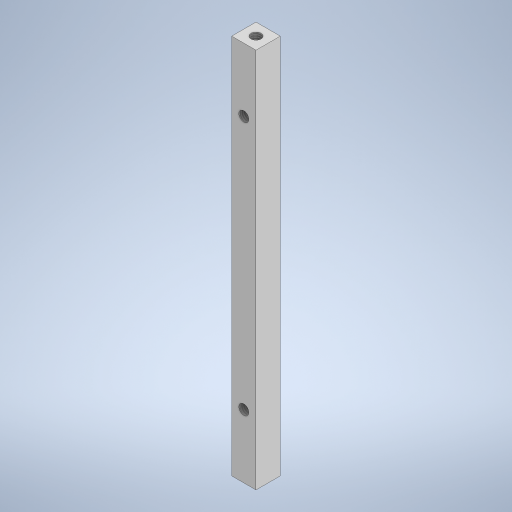
# Autodesk Inventor part: VerticalStrut
Saved by Autodesk Inventor 2023 (Build 270158000, 158)
## iProperties
Created: 2022-07-23
Part Number: VerticalStrut
Material: Generic
Document SubType Name: Modeling
Designer: Aditya Bansal
Density: 1 g/cm^3
Appearance: Default
Author: Aditya Bansal
Autodesk Inventor part; units mm, degrees
ref_plane "YZ Plane" through (0, 0, 0) normal (1, 0, 0) x (0, 1, 0)
ref_plane "XZ Plane" through (0, 0, 0) normal (0, 1, 0) x (-1, 0, 0)
ref_plane "XY Plane" through (0, 0, 0) normal (0, 0, 1) x (1, 0, 0)
sketch "Sketch1" plane through (0, 0, 0) normal (0, 1, 0) x (-1, 0, 0)
  line L0 (0, 0) -> (6, 0)
  line L1 (6, 0) -> (6, -6)
  line L2 (6, -6) -> (0, -6)
  line L3 (0, -6) -> (0, 0)
  dimension "d0" = 6
  constraints: 8 end point, 2 parallel, 2 perpendicular, 1 horizontal
  measures "d0" distance of L0.end L1.end
extrude "Extrusion1" add sketch "Sketch1" along normal blind 47
sketch "Sketch2" plane through (0, 47, 0) normal (0, 1, 0) x (1, 0, 0)
  line L0 (0, 6) -> (-6, 6) projected
  line L1 (0, 0) -> (0, 6) projected
  point P0 (-3, 3)
  point P1 (-3, 6)
  point P2 (0, 3)
  point P3 (-3, 6)
  constraints: 3 midpoint, 1 horizontal alignment, 1 vertical alignment
hole "Hole1" at (-3, 47, -3) direction (0, -1, 0) diameter 2.459 depth 10 tip angle 118 thread size "M3x0.5" class "6H" standard "ANSI Metric M Profile"
sketch "Sketch3" plane through (-6, 47, 0) normal (0, 0, 1) x (1, 0, 0)
  line L0 (0, -47) -> (0, 0) projected
  line L1 (6, -47) -> (6, 0) projected
  line L2 (0, 0) -> (6, 0) projected
  point P0 (3, -47)
  point P1 (3, -15.6667)
  point P2 (0, -94)
  point P3 (6, -94)
  dimension "d17" = 6
  dimension "d18" = 3
  dimension "d19" = 15.6667
  dimension "d20" = 31.3333
  dimension "d21" = 47
  constraints: 1 point on line, 1 vertical alignment
  measures "d17" distance between parallel lines of L0 L1
  measures "d18" distance from line of L1 point (3, -15.667)
  measures "d19" distance from line of point (3, -15.667) L2
  measures "d20" distance of point (3, -15.667) point (3, -47)
  measures "d21" distance from line of L2 point (6, -47)
hole "Hole2" at (-3, 31.3333, 0) direction (0, 0, -1) diameter 2.459 depth 3 tip angle 118 thread size "M3x0.5" class "6H" standard "ANSI Metric M Profile"
sketch "Sketch5" plane through (-6, 0, -6) normal (-1, 0, 0) x (0, 0, 1)
  line L0 (0, 0) -> (6, 0) projected
  point P0 (3, 25)
  point P1 (3, 0)
  dimension "d29" = 25
  constraints: 1 midpoint, 1 vertical alignment
  measures "d29" distance from line of L0 point (3, 25)
hole "Hole3" at (-6, 25, -3) direction (1, 0, 0) diameter 2.459 depth 3 tip angle 118 thread size "M3x0.5" class "6H" standard "ANSI Metric M Profile"
mirror "Mirror2" about plane through (-3, 0, -3) normal (0, -1, 0) of "Extrusion1", "Hole1", "Hole2", "Hole3"
equation "\"d18\" = 0.5 * d17"
equation "\"d19\" = 0.333333 * d21"
equation "\"d20\" = 2 * d19"
body "Solid1"
